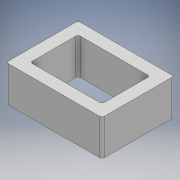
# Autodesk Inventor part: agarose-mold-mouse-brain
Saved by Autodesk Inventor 2017 (Build 210142000, 142)
## iProperties
Created: 2022-08-29
Part Number: agarose-mold-mouse-brain
Material: Generic
Document SubType Name: Modeling
Designer: Nikita
Density: 1 g/cm^3
Appearance: Default
Author: Nikita
Autodesk Inventor part; units mm, degrees
ref_plane "YZ Plane" through (0, 0, 0) normal (1, 0, 0) x (0, 1, 0)
ref_plane "XZ Plane" through (0, 0, 0) normal (0, 1, 0) x (-1, 0, 0)
ref_plane "XY Plane" through (0, 0, 0) normal (0, 0, 1) x (1, 0, 0)
sketch "Sketch1" plane through (0, 0, 0) normal (0, 0, 1) x (1, 0, 0)
  line L0 (15, -10) -> (-15, -10)
  line L1 (-15, -10) -> (-15, 10)
  line L2 (-15, 10) -> (15, 10)
  line L3 (15, 10) -> (15, -10)
  line L4 (15, -10) -> (-15, 10) construction
  line L5 (-15, -10) -> (15, 10) construction
  line L6 (20, -15) -> (-20, -15)
  line L7 (-20, -15) -> (-20, 15)
  line L8 (-20, 15) -> (20, 15)
  line L9 (20, 15) -> (20, -15)
  line L10 (20, -15) -> (-20, 15) construction
  line L11 (-20, -15) -> (20, 15) construction
  point P0 (0, 0)
  dimension "d0" = 30
  dimension "d1" = 20
  dimension "d2" = 40
  dimension "d3" = 30
  constraints: 24 end point, 4 midpoint, 4 parallel, 2 horizontal, 2 perpendicular
  measures "d0" distance of L1.end L2.end
  measures "d1" distance of L0.end L1.end
  measures "d2" distance of L7.end L8.end
  measures "d3" distance of L6.end L7.end
extrude "Extrusion1" add sketch "Sketch1" along normal blind 15
fillet "Fillet1" radius 1 4 edges at (-15, -10, 7.5) (-15, 10, 7.5) (15, 10, 7.5) (15, -10, 7.5)
fillet "Fillet2" radius 1 4 edges at (-20, 15, 7.5) (-20, -15, 7.5) (20, 15, 7.5) (20, -15, 7.5)
body "Solid1"
